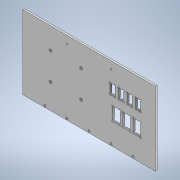
# Autodesk Inventor part: sheetmetalleft2.0
Saved by Autodesk Inventor 2020.2 (Build 242310000, 310)
## iProperties
Created: 2020-02-06
Part Number: sheetmetalleft2.0
Material: Generic
Document SubType Name: Sheet Metal
Designer: ColinP
Density: 1 g/cm^3
Sheet Metal Rule: Default
Appearance: Default
Mass: 83.3891 g
Surface Area: 588.438 cm^2
Volume: 83.3891 cm^3
Author: ColinP
Autodesk Inventor part; units mm, degrees
ref_plane "YZ Plane" through (0, 0, 0) normal (1, 0, 0) x (0, 1, 0)
ref_plane "XZ Plane" through (0, 0, 0) normal (0, 1, 0) x (-1, 0, 0)
ref_plane "XY Plane" through (0, 0, 0) normal (0, 0, 1) x (1, 0, 0)
sketch "Sketch1" plane through (0, 0, 0) normal (0, 0, 1) x (1, 0, 0)
  line L0 (114.3, 63.5) -> (-114.3, 63.5)
  line L1 (-114.3, 63.5) -> (-114.3, -63.5)
  line L2 (-114.3, -63.5) -> (114.3, -63.5)
  line L3 (114.3, -63.5) -> (114.3, 63.5)
  point P0 (0, 0)
  dimension "d0" = 228.6
  dimension "d1" = 127
  measures "d0" distance of L2.end L1.end
  measures "d1" distance of L1.end L0.end
extrude "Plate1" add sketch "Sketch1" along normal blind 3.048
sketch "Sketch2" plane through (0, 0, 3.048) normal (0, 0, 1) x (1, 0, 0)
  line L0 (-114.3, 63.5) -> (-114.3, -63.5) projected
  line L1 (-114.3, -63.5) -> (-114.3, -60.325)
  line L2 (-114.3, -60.325) -> (-76.2, -60.325)
  line L3 (-76.2, -60.325) -> (-38.1, -60.325)
  line L4 (-38.1, -60.325) -> (0, -60.325)
  line L5 (0, -60.325) -> (38.1, -60.325)
  line L6 (38.1, -60.325) -> (76.2, -60.325)
  line L7 (76.2, -60.325) -> (114.3, -60.325)
  line L8 (114.3, -63.5) -> (114.3, 63.5) projected
  point P0 (0, 0)
  dimension "d3" = 3.175
  dimension "d4" = 38.1
  dimension "d5" = 38.1
  dimension "d6" = 38.1
  dimension "d7" = 38.1
  constraints: 14 end point, 7 point on line, 1 perpendicular
  measures "d3" distance of L0.end L1.end
  measures "d4" distance of L1.end L2.end
  measures "d5" distance of L2.end L3.end
  measures "d6" distance of L4.end L5.end
  measures "d7" distance of L5.end L6.end
hole "Hole1" at (-76.2, -60.325, 3.048) at (-38.1, -60.325, 3.048) at (0, -60.325, 3.048) at (38.1, -60.325, 3.048) at (76.2, -60.325, 3.048) direction (0, 0, -1) diameter 3.2766 depth 3.048 clearance for "Hex Machine Screw" size "#4" standard "Ansi Unified Screw Threads"
sketch "Sketch3" plane through (0, 0, 3.048) normal (0, 0, 1) x (1, 0, 0)
  line L0 (-114.3, -63.5) -> (114.3, -63.5) projected
  line L1 (-114.3, -63.5) -> (-114.3, -25.4)
  line L2 (-114.3, -63.5) -> (-114.3, 63.5) projected
  line L3 (-114.3, -25.4) -> (-88.9, -25.4)
  line L4 (-88.9, -25.4) -> (-88.9, 31.6)
  line L5 (-88.9, 31.6) -> (-43.9, 31.6)
  line L6 (-43.9, 31.6) -> (-43.9, -25.4)
  line L7 (-43.9, -25.4) -> (-88.9, -25.4)
  line L8 (-66.4, -25.4) -> (-66.4, -20.4)
  line L9 (-66.4, 31.6) -> (-66.4, 26.6)
  line L10 (-43.9, 31.6) -> (-36.28, 31.6)
  line L11 (-36.28, 31.6) -> (-36.28, -25.4)
  line L12 (-36.28, -25.4) -> (8.72, -25.4)
  line L13 (8.72, -25.4) -> (8.72, 31.6)
  line L14 (8.72, 31.6) -> (-36.28, 31.6)
  line L15 (-13.78, 31.6) -> (-13.78, 26.6)
  line L16 (-13.78, -25.4) -> (-13.78, -20.4)
  point P0 (0, 0)
  dimension "d15" = 38.1
  dimension "d16" = 25.4
  dimension "d17" = 57
  dimension "d18" = 45
  dimension "d19" = 5
  dimension "d20" = 5
  dimension "d21" = 7.62
  dimension "d22" = 45
  dimension "d23" = 5
  dimension "d24" = 5
  constraints: 30 end point, 9 perpendicular, 4 midpoint, 4 vertical, 3 point on line, 1 horizontal
  measures "d15" distance of L0.start L1.end
  measures "d16" distance of L1.end L3.end
  measures "d17" distance of L3.end L4.end
  measures "d18" distance of L4.end L5.end
  measures "d19" distance of L8.start L8.end
  measures "d20" distance of L9.start L9.end
  measures "d21" distance of L5.end L10.end
  measures "d22" distance of L11.end L12.end
  measures "d23" distance of L15.start L15.end
  measures "d24" distance of L16.start L16.end
hole "Hole2" at (-66.4, 26.6, 3.048) at (-13.78, 26.6, 3.048) at (-13.78, -20.4, 3.048) at (-66.4, -20.4, 3.048) direction (0, 0, -1) diameter 4.4958 depth 3.048 clearance for "Hex Machine Screw" size "#8" standard "Ansi Unified Screw Threads"
sketch "Sketch4" plane through (0, 0, 3.048) normal (0, 0, 1) x (1, 0, 0)
  line L0 (-114.3, -63.5) -> (114.3, -63.5) projected
  line L1 (114.3, -63.5) -> (114.3, -25.4)
  line L2 (114.3, -63.5) -> (114.3, 63.5) projected
  line L3 (114.3, -25.4) -> (88.9, -25.4)
  line L4 (88.9, -25.4) -> (88.9, -2.794)
  line L5 (88.9, -2.794) -> (76.2, -2.794)
  line L6 (76.2, -2.794) -> (71.12, -2.794)
  line L7 (71.12, -2.794) -> (58.42, -2.794)
  line L8 (58.42, -2.794) -> (53.34, -2.794)
  line L9 (53.34, -2.794) -> (40.64, -2.794)
  line L10 (40.64, -2.794) -> (40.64, -25.4)
  line L11 (40.64, -25.4) -> (53.34, -25.4)
  line L12 (53.34, -25.4) -> (53.34, -2.794)
  line L13 (58.42, -2.794) -> (58.42, -25.4)
  line L14 (58.42, -25.4) -> (71.12, -25.4)
  line L15 (71.12, -25.4) -> (71.12, -2.794)
  line L16 (76.2, -2.794) -> (76.2, -25.4)
  line L17 (76.2, -25.4) -> (88.9, -25.4)
  point P0 (0, 0)
  dimension "d32" = 38.1
  dimension "d33" = 25.4
  dimension "d34" = 22.606
  dimension "d35" = 12.7
  dimension "d36" = 5.08
  dimension "d37" = 12.7
  dimension "d38" = 5.08
  dimension "d39" = 12.7
  constraints: 32 end point, 8 point on line, 7 perpendicular, 2 parallel, 1 vertical
  measures "d32" distance of L0.end L1.end
  measures "d33" distance of L1.end L3.end
  measures "d34" distance of L3.end L4.end
  measures "d35" distance of L4.end L5.end
  measures "d36" distance of L5.end L6.end
  measures "d37" distance of L6.end L7.end
  measures "d38" distance of L7.end L8.end
  measures "d39" distance of L8.end L9.end
extrude "Cut1" cut sketch "Sketch4" against normal blind 3.048
sketch "Sketch5" plane through (0, 0, 3.048) normal (0, 0, 1) x (1, 0, 0)
  line L0 (-114.3, -63.5) -> (114.3, -63.5) projected
  line L1 (114.3, -63.5) -> (114.3, 12.7)
  line L2 (114.3, -63.5) -> (114.3, 63.5) projected
  line L3 (114.3, 12.7) -> (88.9, 12.7)
  line L4 (88.9, 12.7) -> (80.518, 12.7)
  line L5 (80.518, 12.7) -> (80.518, 29.718)
  line L6 (80.518, 29.718) -> (74.168, 29.718)
  line L7 (74.168, 29.718) -> (74.168, 12.7)
  line L8 (74.168, 12.7) -> (65.786, 12.7)
  line L9 (65.786, 12.7) -> (65.786, 29.718)
  line L10 (65.786, 29.718) -> (74.168, 29.718)
  line L11 (80.518, 29.718) -> (88.9, 29.718)
  line L12 (88.9, 29.718) -> (88.9, 12.7)
  line L13 (65.786, 29.718) -> (59.436, 29.718)
  line L14 (59.436, 29.718) -> (59.436, 12.7)
  line L15 (59.436, 12.7) -> (51.054, 12.7)
  line L16 (51.054, 12.7) -> (51.054, 29.718)
  line L17 (51.054, 29.718) -> (59.436, 29.718)
  line L18 (51.054, 29.718) -> (44.704, 29.718)
  line L19 (44.704, 29.718) -> (44.704, 12.7)
  line L20 (44.704, 12.7) -> (36.322, 12.7)
  line L21 (36.322, 12.7) -> (36.322, 29.718)
  line L22 (36.322, 29.718) -> (44.704, 29.718)
  point P0 (0, 0)
  dimension "d42" = 76.2
  dimension "d43" = 25.4
  dimension "d44" = 270
  dimension "d45" = 8.382
  dimension "d46" = 17.018
  dimension "d47" = 6.35
  dimension "d48" = 8.382
  dimension "d49" = 6.35
  dimension "d50" = 8.382
  dimension "d51" = 6.35
  dimension "d52" = 8.382
  constraints: 42 end point, 13 point on line, 12 perpendicular, 1 collinear, 1 horizontal
  measures "d42" distance of L0.end L1.end
  measures "d43" distance of L1.end L3.end
  measures "d45" distance of L3.end L4.end
  measures "d46" distance of L4.end L5.end
  measures "d47" distance of L5.end L6.end
  measures "d48" distance of L7.end L8.end
  measures "d49" distance of L9.end L13.end
  measures "d50" distance of L14.end L15.end
  measures "d51" distance of L16.end L18.end
  measures "d52" distance of L19.end L20.end
extrude "Cut2" cut sketch "Sketch5" against normal blind 3.048
sketch "Sketch6" plane through (0, 0, 3.048) normal (0, 0, 1) x (1, 0, 0)
  line L0 (-114.3, 63.5) -> (114.3, 63.5) projected
  line L1 (-114.3, 63.5) -> (-114.3, 50.8)
  line L2 (-114.3, 63.5) -> (-114.3, -63.5) projected
  line L3 (-114.3, 50.8) -> (-38.1, 50.8)
  line L4 (-38.1, 50.8) -> (38.1, 50.8)
  line L5 (38.1, 50.8) -> (114.246, 50.8)
  point P0 (0, 0)
  dimension "d55" = 12.7
  dimension "d56" = 76.2
  dimension "d57" = 76.2
  constraints: 8 end point, 3 point on line, 1 perpendicular
  measures "d55" distance of L0.start L1.end
  measures "d56" distance of L1.end L3.end
  measures "d57" distance of L3.end L4.end
hole "Hole3" at (-38.1, 50.8, 3.048) at (38.1, 50.8, 3.048) direction (0, 0, -1) diameter 2.1565 depth 8.8646 thread size "4-40 UNC" class "2B" standard "ANSI Unified Screw Threads"
sketch "Sketch7" plane through (0, 0, 0) normal (0, 0, -1) x (-1, 0, 0)
  circle A0 centre (38.1, 50.8) radius 1.0782 projected
  circle A1 centre (-38.1, 50.8) radius 1.0782 projected
  line L0 (-65.786, 29.718) -> (-65.786, 12.7) projected
  line L1 (-65.786, 12.7) -> (-74.168, 12.7) projected
  line L2 (-74.168, 12.7) -> (-74.168, 29.718) projected
  line L3 (-74.168, 29.718) -> (-65.786, 29.718) projected
  line L4 (-36.322, 29.718) -> (-36.322, 12.7) projected
  line L5 (-36.322, 12.7) -> (-44.704, 12.7) projected
  line L6 (-44.704, 12.7) -> (-44.704, 29.718) projected
  line L7 (-44.704, 29.718) -> (-36.322, 29.718) projected
  line L8 (-51.054, 29.718) -> (-51.054, 12.7) projected
  line L9 (-51.054, 12.7) -> (-59.436, 12.7) projected
  line L10 (-59.436, 12.7) -> (-59.436, 29.718) projected
  line L11 (-59.436, 29.718) -> (-51.054, 29.718) projected
  line L12 (-88.9, 29.718) -> (-80.518, 29.718) projected
  line L13 (-80.518, 29.718) -> (-80.518, 12.7) projected
  line L14 (-80.518, 12.7) -> (-88.9, 12.7) projected
  line L15 (-88.9, 12.7) -> (-88.9, 29.718) projected
  line L16 (-58.42, -2.794) -> (-58.42, -25.4) projected
  line L17 (-58.42, -25.4) -> (-71.12, -25.4) projected
  line L18 (-71.12, -25.4) -> (-71.12, -2.794) projected
  line L19 (-71.12, -2.794) -> (-58.42, -2.794) projected
  line L20 (-40.64, -2.794) -> (-40.64, -25.4) projected
  line L21 (-40.64, -25.4) -> (-53.34, -25.4) projected
  line L22 (-53.34, -25.4) -> (-53.34, -2.794) projected
  line L23 (-53.34, -2.794) -> (-40.64, -2.794) projected
  line L24 (-88.9, -2.794) -> (-76.2, -2.794) projected
  line L25 (-76.2, -2.794) -> (-76.2, -25.4) projected
  line L26 (-76.2, -25.4) -> (-88.9, -25.4) projected
  line L27 (-88.9, -25.4) -> (-88.9, -2.794) projected
  circle A2 centre (13.78, -20.4) radius 2.2479 projected
  circle A3 centre (66.4, 26.6) radius 2.2479 projected
  circle A4 centre (13.78, 26.6) radius 2.2479 projected
  circle A5 centre (66.4, -20.4) radius 2.2479 projected
  circle A6 centre (-38.1, -60.325) radius 1.6383 projected
  circle A7 centre (38.1, -60.325) radius 1.6383 projected
  circle A8 centre (76.2, -60.325) radius 1.6383 projected
  circle A9 centre (0, -60.325) radius 1.6383 projected
  circle A10 centre (-76.2, -60.325) radius 1.6383 projected
  line L28 (-114.3, 63.5) -> (114.3, 63.5) projected
  line L29 (-114.3, -63.5) -> (-114.3, 63.5) projected
  line L30 (114.3, -63.5) -> (-114.3, -63.5) projected
  line L31 (114.3, 63.5) -> (114.3, -63.5) projected
  point P0 (0, 0)
hole "Hole4" at (40.64, -2.794, 0) at (40.64, -25.4, 0) at (53.34, -25.4, 0) at (53.34, -2.794, 0) at (58.42, -2.794, 0) at (58.42, -25.4, 0) at (71.12, -25.4, 0) at (71.12, -2.794, 0) at (76.2, -2.794, 0) at (76.2, -25.4, 0) at (88.9, -25.4, 0) at (88.9, -2.794, 0) at (80.518, 29.718, 0) at (88.9, 29.718, 0) at (88.9, 12.7, 0) at (80.518, 12.7, 0) at (74.168, 12.7, 0) at (74.168, 29.718, 0) at (65.786, 29.718, 0) at (65.786, 12.7, 0) at (59.436, 12.7, 0) at (59.436, 29.718, 0) at (51.054, 29.718, 0) at (51.054, 12.7, 0) at (44.704, 12.7, 0) at (36.322, 12.7, 0) at (36.322, 29.718, 0) at (44.704, 29.718, 0) direction (0, 0, 1) diameter 2.794 depth 3.048 clearance for "Flat Head Machine Screw (82)" size "#3" standard "Ansi Unified Screw Threads"
equation "\"d13\" = Thickness"
equation "\"d30\" = Thickness"
equation "\"d40\" = Thickness"
equation "\"d53\" = Thickness"
equation "\"d70\" = Thickness"
equation "\"d2\" = Thickness"
equation "\"BendRadius\" = Thickness"
equation "\"BendReliefWidth\" = Thickness"
equation "\"BendReliefDepth\" = 0.5 * Thickness"
equation "\"CornerReliefSize\" = 4 * Thickness"
equation "\"MinimumRemnant\" = 2 * Thickness"
equation "\"TransitionRadius\" = BendRadius"
equation "\"JacobiRadiusSize\" = BendRadius"
equation "\"GapSize\" = Thickness"
equation "\"Thickness\" = 3.048"
body "Solid1"
